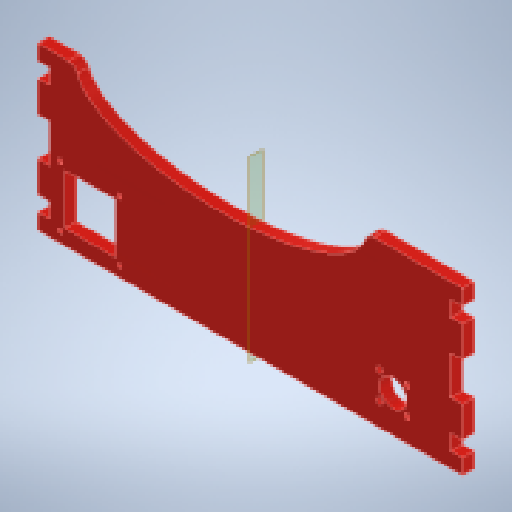
# Autodesk Inventor part: боковая стенка
Saved by Autodesk Inventor 2024.2 (Build 282272000, 272)
## iProperties
Created: 2025-11-20
Part Number: боковая стенка
Material: Типовые
Document SubType Name: Modeling
Designer: Zakhar
Density: 1 g/cm^3
Appearance: Оранжево-красный
Mass: 81.5682 g
Surface Area: 329.882 cm^2
Volume: 81.5682 cm^3
Author: Zakhar
Autodesk Inventor part; units mm, degrees
ref_plane "YZ Plane" through (0, 0, 0) normal (1, 0, 0) x (0, 1, 0)
ref_plane "XZ Plane" through (0, 0, 0) normal (0, 1, 0) x (-1, 0, 0)
ref_plane "XY Plane" through (0, 0, 0) normal (0, 0, 1) x (1, 0, 0)
sketch "Эскиз1" plane through (0, 0, 0) normal (0, 0, 1) x (1, 0, 0)
  line L0 (220, 84) -> (220, 0)
  line L1 (220, 0) -> (0, 0)
  line L2 (0, 0) -> (0, 84)
  line L3 (6, 0) -> (0, 0)
  line L4 (0, 76) -> (6, 76)
  line L5 (6, 76) -> (6, 8)
  line L6 (6, 8) -> (0, 8)
  line L7 (0, 8) -> (0, 76)
  ellipse E0 centre (95, 84) end of major axis (170, 84) minor radius 28.3094 (20, 84) -> (170, 84) ccw
  line L8 (0, 84) -> (20, 84)
  line L9 (170, 84) -> (220, 84)
  line L10 (220, 76) -> (214, 76)
  line L11 (214, 76) -> (214, 8)
  line L12 (214, 8) -> (220, 8)
  line L13 (220, 8) -> (220, 76)
  line L14 (0, 68) -> (6, 68)
  line L15 (6, 68) -> (6, 52)
  line L16 (6, 52) -> (0, 52)
  line L17 (0, 52) -> (0, 68)
  line L18 (0, 32) -> (6, 32)
  line L19 (6, 32) -> (6, 16)
  line L20 (6, 16) -> (0, 16)
  line L21 (0, 16) -> (0, 32)
  line L22 (214, 68) -> (220, 68)
  line L23 (214, 52) -> (220, 52)
  line L24 (214, 32) -> (220, 32)
  line L25 (214, 16) -> (220, 16)
  point P0 (217, 8)
  point P1 (220, 8)
  point P2 (3, 76)
  point P3 (3, 0)
  point P4 (217, 76)
  point P5 (3, 68)
  point P6 (0, 16)
  point P7 (0, 52)
  point P8 (217, 68)
  point P9 (217, 32)
  point P10 (217, 16)
  point P11 (217, 52)
  point P12 (220, 32)
  point P13 (220, 52)
  point P14 (220, 68)
  dimension "d1" = 75
  dimension "d0" = 220
  dimension "d2" = 125
  dimension "d3" = 84
  dimension "d4" = 150
  dimension "d5" = 84
  dimension "d6" = 6
  dimension "d7" = 8
  dimension "d10" = 6
  dimension "d11" = 8
  dimension "d12" = 8
  dimension "d13" = 8
  dimension "d14" = 84
  dimension "d35" = 8
  dimension "d36" = 8
  dimension "d37" = 16
  dimension "d38" = 16
  dimension "d39" = 8
  dimension "d40" = 8
  dimension "d41" = 16
  dimension "d42" = 16
  constraints: 52 end point, 13 point on line, 11 parallel, 10 perpendicular, 9 midpoint, 6 horizontal, 2 collinear, 1 coincident, 4 other
  measures "d0" distance of L1.start L1.end
  measures "d2" distance of L0.start point (95, 84)
  measures "d3" distance between parallel lines of L1 L9
  measures "d4" distance of L8.end L9.start
  measures "d5" distance from line of L1 point (95, 84)
  measures "d6" distance of L13.end L11.start
  measures "d7" vertical distance of point (217, 8) L1.start
  measures "d10" distance between parallel lines of L2 L5
  measures "d11" distance from line of L8 point (3, 76)
  measures "d12" distance from line of point (3, 0) L6
  measures "d13" distance from line of L9 point (217, 76)
  measures "d14" distance between parallel lines of L1 L8
  measures "d35" distance between parallel lines of L20 L6
  measures "d36" distance between parallel lines of L4 L14
  measures "d37" distance between parallel lines of L18 L20
  measures "d38" distance from line of point (3, 68) L16
  measures "d39" distance from line of L10 point (217, 68)
  measures "d40" distance from line of L25 point (217, 8)
  measures "d41" distance of point (217, 32) point (217, 16)
  measures "d42" distance of point (217, 68) point (217, 52)
extrude "Выдавливание1" add sketch "Эскиз1" along normal blind 6 contours L0 L10 L11 L12 L1 L2 L6 L5 L4 L8 E0 L9 | L0 L23 L11 L22 | L0 L25 L11 L24 | L14 L5 L16 L2 | L18 L5 L20 L2
sketch "Эскиз2" plane through (0, 0, 6) normal (0, 0, 1) x (1, 0, 0)
  line L0 (0, 0) -> (220, 0) projected
  line L1 (6, 0) -> (48, 0)
  line L2 (48, 0) -> (48, 8)
  line L3 (48, 8) -> (6, 8)
  line L4 (6, 8) -> (6, 0)
  line L5 (48, 0) -> (40, 0)
  line L6 (40, 0) -> (40, 42)
  line L7 (40, 42) -> (48, 42)
  line L8 (48, 42) -> (48, 0)
  line L9 (48, 42) -> (6, 42)
  line L10 (6, 42) -> (6, 34)
  line L11 (6, 34) -> (48, 34)
  line L12 (48, 34) -> (48, 42)
  line L13 (6, 42) -> (14, 42)
  line L14 (14, 42) -> (14, 0)
  line L15 (14, 0) -> (6, 0)
  line L16 (6, 0) -> (6, 42)
  line L17 (6, 16) -> (6, 8) projected
  circle A0 centre (11.5, 36.5) radius 1.5
  circle A1 centre (42.5, 36.5) radius 1.5
  circle A2 centre (42.5, 5.5) radius 1.5
  circle A3 centre (11.5, 5.5) radius 1.5
  circle A4 centre (184, 19) radius 7
  circle A5 centre (177, 25.9159) radius 1.5
  circle A6 centre (191, 26.0852) radius 1.5
  circle A7 centre (191, 12) radius 1.5
  circle A8 centre (177, 12) radius 1.5
  line L18 (177, 42.7055) -> (177, 0) construction
  line L19 (173.1146, 12) -> (210.5161, 12) construction
  line L20 (0, 0) -> (220, 0) projected
  line L21 (174.3072, 25.8833) -> (201.7049, 26.2146) construction
  line L22 (191, 29.1476) -> (191, 5.5) construction
  line L23 (214, 8) -> (214, 16) projected
  circle A9 centre (27, 21) radius 12.5
  point P0 (27, 0)
  point P1 (6, 76)
  point P2 (14, 34)
  point P3 (14, 8)
  point P4 (40, 8)
  point P5 (40, 34)
  dimension "d15" = 42
  dimension "d16" = 42
  dimension "d17" = 8
  dimension "d18" = 8
  dimension "d19" = 8
  dimension "d20" = 8
  dimension "d21" = 3
  dimension "d22" = 3
  dimension "d23" = 3
  dimension "d24" = 3
  dimension "d25" = 5.5
  dimension "d26" = 5.5
  dimension "d27" = 5.5
  dimension "d28" = 5.5
  dimension "d29" = 5.5
  dimension "d30" = 5.5
  dimension "d31" = 5.5
  dimension "d32" = 5.5
  dimension "d78" = 14
  dimension "d80" = 3
  dimension "d81" = 3
  dimension "d82" = 3
  dimension "d83" = 3
  dimension "d91" = 30
  dimension "d93" = 21
  dimension "d94" = 21
  dimension "d95" = 25
  constraints: 40 end point, 12 point on line, 10 centre point, 8 parallel, 5 horizontal, 4 perpendicular, 4 tangent, 2 vertical, 1 collinear, 1 midpoint, 1 other
  measures "d15" distance of L10.end L11.end
  measures "d16" distance of L15.end L9.end
  measures "d17" distance between parallel lines of L9 L11
  measures "d18" distance between parallel lines of L8 L6
  measures "d19" distance from line of point (27, 0) L3
  measures "d20" distance between parallel lines of L16 L14
  measures "d21" diameter of A0
  measures "d22" diameter of A1
  measures "d23" diameter of A2
  measures "d24" diameter of A3
  measures "d25" distance from line of L1 A3.centre
  measures "d26" distance from line of L16 A3.centre
  measures "d27" distance from line of L8 A2.centre
  measures "d28" distance from line of L0 A2.centre
  measures "d29" distance from line of L12 A1.centre
  measures "d30" distance from line of L7 A1.centre
  measures "d31" distance from line of L9 A0.centre
  measures "d32" distance from line of L10 A0.centre
  measures "d78" diameter of A4
  measures "d80" diameter of A5
  measures "d81" diameter of A6
  measures "d82" diameter of A7
  measures "d83" diameter of A8
  measures "d91" distance from line of L23 A4.centre
  measures "d93" distance of point (27, 0) A9.centre
  measures "d94" distance from line of L16 A9.centre
  measures "d95" diameter of A9
extrude "Выдавливание2" cut sketch "Эскиз2" against normal blind 6 contours A0 | A1 | A2 | A3 | A4 | A5 | A6 | A7 | A8 | A9
ref_plane "РабПлоскость1" through (110, 8, 0) normal (-1, 0, 0) x (0, 0, 1)
sketch "Эскиз5" plane through (0, 0, 0) normal (0, -1, 0) x (1, 0, 0)
  circle A0 centre (115, 3) radius 1.5
  circle A1 centre (105, 3) radius 1.5
  line L0 (110, -1.2) -> (110, 7.2) projected
  line L1 (0, 0) -> (220, 0) projected
  dimension "d70" = 5
  dimension "d71" = 5
  dimension "d72" = 3
  dimension "d73" = 3
  dimension "d74" = 3
  dimension "d75" = 3
  constraints: 2 centre point
  measures "d70" distance from line of L0 A1.centre
  measures "d71" distance from line of L0 A0.centre
  measures "d72" distance from line of L1 A0.centre
  measures "d73" distance from line of L1 A1.centre
  measures "d74" diameter of A1
  measures "d75" diameter of A0
extrude "Выдавливание3" cut sketch "Эскиз5" against normal blind 6
fillet "Сопряжение1" radius 5 2 edges at (170, 84, 3) (20, 84, 3)
equation "\"d36\" = d35"
equation "\"d38\" = d37"
equation "\"d40\" = d39"
equation "\"d42\" = d41"
equation "\"d22\" = d21"
equation "\"d23\" = d21"
equation "\"d24\" = d21"
